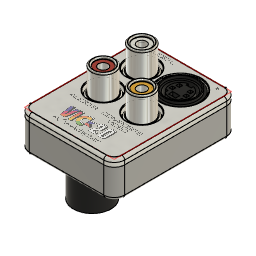
VIC-20_AV_Adapter_case v2 v2 (Autodesk Fusion 360 design; units mm, degrees)
Autodesk Fusion 360 part; units mm, degrees
(part 1 of 2)
sketch "top place" plane through (0, 0, 0) normal (0, 0, 1) x (1, 0, 0) in component "PCB"
  line L0 (0, 1) -> (0, 37)
  circle A0 centre (7, 32) radius 1.7
  arc A1 (23.4749, 22.3133) -> (18.5251, 22.3133) centre (21, 18) ccw
  arc A2 (3.4645, 34.2627) -> (3.4645, 29.7373) centre (7, 32) ccw
  circle A3 centre (21, 18) radius 3.1
  arc A4 (11.3133, 29.5251) -> (11.3133, 34.4749) centre (7, 32) ccw
  arc A5 (16.6867, 20.4749) -> (16.6867, 15.5251) centre (21, 18) ccw
  arc A6 (24.5355, 15.7373) -> (24.5355, 20.2627) centre (21, 18) ccw
  arc A7 (4.5251, 27.6867) -> (9.4749, 27.6867) centre (7, 32) ccw
  arc A8 (11.3133, 15.5251) -> (11.3133, 20.4749) centre (7, 18) ccw
  arc A9 (4.5251, 13.6867) -> (9.4749, 13.6867) centre (7, 18) ccw
  arc A10 (2.6867, 34.4749) -> (2.6867, 29.5251) centre (7, 32) ccw
  arc A11 (10.5355, 29.7373) -> (10.5355, 34.2627) centre (7, 32) ccw
  arc A12 (17.4645, 20.2627) -> (17.4645, 15.7373) centre (21, 18) ccw
  circle A13 centre (7, 18) radius 1.7
  arc A14 (9.2627, 21.5355) -> (4.7373, 21.5355) centre (7, 18) ccw
  arc A15 (4.7373, 21.5355) -> (3.4645, 20.2627) centre (7, 18) ccw
  arc A16 (10.5355, 20.2627) -> (9.2627, 21.5355) centre (7, 18) ccw
  arc A17 (17.4645, 15.7373) -> (18.7373, 14.4645) centre (21, 18) ccw
  arc A18 (2.6867, 29.5251) -> (4.5251, 27.6867) centre (7, 32) ccw
  arc A19 (18.5251, 22.3133) -> (16.6867, 20.4749) centre (21, 18) ccw
  arc A20 (3.4645, 29.7373) -> (4.7373, 28.4645) centre (7, 32) ccw
  arc A21 (18.7373, 21.5355) -> (17.4645, 20.2627) centre (21, 18) ccw
  arc A22 (11.3133, 20.4749) -> (9.4749, 22.3133) centre (7, 18) ccw
  arc A23 (9.2627, 28.4645) -> (10.5355, 29.7373) centre (7, 32) ccw
  arc A24 (9.4749, 13.6867) -> (11.3133, 15.5251) centre (7, 18) ccw
  arc A25 (24.5355, 20.2627) -> (23.2627, 21.5355) centre (21, 18) ccw
  arc A26 (4.5251, 36.3133) -> (2.6867, 34.4749) centre (7, 32) ccw
  arc A27 (3.4645, 15.7373) -> (4.7373, 14.4645) centre (7, 18) ccw
  line L1 (0, 1) -> (0, 38)
  arc A28 (1, 39) -> (0, 38) centre (1, 38) ccw
  arc A29 (29, 38) -> (28, 39) centre (28, 38) ccw
  arc A30 (0, 1) -> (1, 0) centre (1, 1) ccw
  line L2 (28, 0) -> (1, 0)
  line L3 (29, 38) -> (29, 1)
  line L4 (1, 39) -> (28, 39)
  arc A31 (28, 0) -> (29, 1) centre (28, 1) ccw
  circle A32 centre (21, 18) radius 1.7
  arc A33 (9.4749, 36.3133) -> (4.5251, 36.3133) centre (7, 32) ccw
  arc A34 (25.3133, 15.5251) -> (25.3133, 20.4749) centre (21, 18) ccw
  arc A35 (18.5251, 13.6867) -> (23.4749, 13.6867) centre (21, 18) ccw
  arc A36 (18.7373, 14.4645) -> (23.2627, 14.4645) centre (21, 18) ccw
  arc A37 (9.2627, 35.5355) -> (4.7373, 35.5355) centre (7, 32) ccw
  arc A38 (3.4645, 20.2627) -> (3.4645, 15.7373) centre (7, 18) ccw
  line L5 (19.7, 30.5) -> (19.7, 29)
  arc A39 (4.7373, 28.4645) -> (9.2627, 28.4645) centre (7, 32) ccw
  line L6 (21.9, 35) -> (21.9, 35.8)
  circle A40 centre (7, 32) radius 3.1
  line L7 (22.9, 32.2) -> (23.4, 32.2)
  line L8 (20.1, 35) -> (20.1, 35.8)
  arc A41 (9.4749, 22.3133) -> (4.5251, 22.3133) centre (7, 18) ccw
  line L9 (22.3, 29) -> (22.3, 30.5)
  circle A42 centre (7, 18) radius 3.1
  arc A43 (4.7373, 14.4645) -> (9.2627, 14.4645) centre (7, 18) ccw
  arc A44 (10.5355, 15.7373) -> (10.5355, 20.2627) centre (7, 18) ccw
  arc A45 (2.6867, 20.4749) -> (2.6867, 15.5251) centre (7, 18) ccw
  arc A46 (23.2627, 21.5355) -> (18.7373, 21.5355) centre (21, 18) ccw
  line L10 (22.3, 30.5) -> (19.7, 30.5)
  line L11 (19.6, 33) -> (19.6, 34.2)
  line L12 (22.4, 33) -> (22.8, 33)
  line L13 (19.6, 34.2) -> (19.2, 34.2)
  line L14 (19.6, 33) -> (19.2, 33)
  arc A47 (16.2, 31) -> (25.8, 31) centre (21, 32.05) ccw
  arc A48 (25.8, 33) -> (16.2, 33) centre (21, 32) ccw
  line L15 (1.1113, 7.3025) -> (1.4287, 7.62)
  line L16 (3.6513, 8.5725) -> (3.3338, 8.255)
  line L17 (19.1, 32.2) -> (19.1, 31)
  line L18 (20.1, 35) -> (21.9, 35)
  line L19 (3.6513, 7.3025) -> (3.6513, 5.3975)
  line L20 (22.4, 34.2) -> (22.4, 33)
  line L21 (22.9, 31) -> (23.4, 31)
  line L22 (22.4, 34.2) -> (22.8, 34.2)
  line L23 (19.1, 32.2) -> (18.6, 32.2)
  line L24 (19.7, 29) -> (22.3, 29)
  line L25 (22.9, 31) -> (22.9, 32.2)
  line L26 (19.1, 31) -> (18.6, 31)
  circle A49 centre (21, 32) radius 5.6
  line L27 (3.0163, 5.3975) -> (3.6513, 5.3975)
  line L28 (3.6513, 9.8425) -> (3.6513, 8.5725)
  line L29 (1.1113, 6.0325) -> (1.7463, 5.3975)
  line L30 (1.1113, 8.5725) -> (1.1113, 9.8425)
  line L31 (1.1113, 6.0325) -> (1.1113, 7.3025)
  circle A50 centre (21, 32) radius 6
  line L32 (3.0163, 10.4775) -> (3.6513, 9.8425)
  line L33 (3.3338, 7.62) -> (3.6513, 7.3025)
  line L34 (1.7463, 10.4775) -> (3.0163, 10.4775)
  line L35 (1.4287, 8.255) -> (1.1113, 8.5725)
  circle A51 centre (21, 32) radius 6.9
  line L36 (1.7463, 5.3975) -> (3.0163, 5.3975)
  line L37 (1.1113, 9.8425) -> (1.7463, 10.4775)
  line L38 (23.6, 34.2) -> (23.6, 33)
  line L39 (2.6353, 6.4135) -> (2.6353, 6.9215)
  line L40 (17.9, 32.2) -> (17.9, 31)
  arc A52 (25.3133, 20.4749) -> (23.4749, 22.3133) centre (21, 18) ccw
  arc A53 (9.4749, 27.6867) -> (11.3133, 29.5251) centre (7, 32) ccw
  arc A54 (23.2627, 14.4645) -> (24.5355, 15.7373) centre (21, 18) ccw
  line L41 (24.1, 31) -> (24.1, 32.2)
  arc A55 (23.4749, 13.6867) -> (25.3133, 15.5251) centre (21, 18) ccw
  arc A56 (11.3133, 34.4749) -> (9.4749, 36.3133) centre (7, 32) ccw
  line L42 (18.6, 32.2) -> (17.9, 32.2)
  line L43 (22.8, 34.2) -> (23.6, 34.2)
  line L44 (2.6353, 8.9535) -> (2.6353, 9.4615)
  line L45 (2.6353, 9.4615) -> (2.1273, 9.4615)
  line L46 (23.6, 33) -> (22.8, 33)
  arc A57 (4.7373, 35.5355) -> (3.4645, 34.2627) centre (7, 32) ccw
  arc A58 (16.6867, 15.5251) -> (18.5251, 13.6867) centre (21, 18) ccw
  arc A59 (10.5355, 34.2627) -> (9.2627, 35.5355) centre (7, 32) ccw
  arc A60 (2.6867, 15.5251) -> (4.5251, 13.6867) centre (7, 18) ccw
  arc A61 (16.2, 33) -> (16.2, 31) centre (21, 32) ccw
  line L47 (17.9, 31) -> (18.6, 31)
  arc A62 (4.5251, 22.3133) -> (2.6867, 20.4749) centre (7, 18) ccw
  line L48 (23.4, 31) -> (24.1, 31)
  line L49 (19.2, 34.2) -> (18.4, 34.2)
  line L50 (18.4, 33) -> (19.2, 33)
  line L51 (24.1, 32.2) -> (23.4, 32.2)
  line L52 (18.4, 34.2) -> (18.4, 33)
  arc A63 (9.2627, 14.4645) -> (10.5355, 15.7373) centre (7, 18) ccw
  arc A64 (25.8, 31) -> (25.8, 33) centre (21, 32) ccw
  line L53 (1.7463, 7.9375) -> (1.4287, 8.255)
  line L54 (2.1273, 8.9535) -> (2.6353, 8.9535)
  line L55 (3.0163, 7.9375) -> (3.3338, 7.62)
  line L56 (2.1273, 6.4135) -> (2.6353, 6.4135)
  line L57 (2.1273, 9.4615) -> (2.1273, 8.9535)
  line L58 (2.1273, 6.9215) -> (2.1273, 6.4135)
  line L59 (2.6353, 6.9215) -> (2.1273, 6.9215)
  line L60 (1.7463, 7.9375) -> (3.0163, 7.9375)
  line L61 (1.4287, 7.62) -> (1.7463, 7.9375)
  line L62 (3.3338, 8.255) -> (3.0163, 7.9375)
  circle A65 centre (21, 32) radius 4.9031
  line L63 (17.6459, 30) -> (18.5, 30)
  line L64 (20.0999, 35.8) -> (20.1, 35)
  line L65 (20.1, 35) -> (21.9, 35)
  line L66 (21.9, 35) -> (21.9, 35.8)
  circle A66 centre (21, 32) radius 3.9051
  line L67 (18.5, 30) -> (18.5, 29)
  line L68 (23.5, 30) -> (24.3541, 30)
  line L69 (23.5, 30) -> (23.5, 29)
  constraint concentric A48 A65
  constraint equal A48 A65
  constraint perpendicular L6 L65
  constraint coincident L6.end A66
  constraint coincident L63.start A66
  constraint coincident A66 L67.end
  constraint perpendicular L63 L67
  constraint coincident A66 L68.end
  constraint coincident A66 L69.end
  constraint perpendicular L68 L69
extrude "Extrude1" add sketch "top place" against normal blind 1.6 contours L0 L1 A28 A29 A30 L2 L3 L4 A31 | A0 | A1 A5 A19 A34 A35 A52 A55 A58 | A2 A11 A20 A23 A37 A39 A57 A59 | A3 | A4 A7 A10 A18 A26 A33 A53 A56 | A6 A12 A17 A21 A25 A36 A46 A54 | A8 A9 A22 A24 A41 A45 A60 A62 | A13 | A14 A15 A16 A27 A38 A43 A44 A63 | A32 | L5 L9 L10 L24 | L6 L8 L18 L64 L65 L66 A66 | L6 L8 L18 L63 L64 L65 L66 A66 L67 L68 L69 | A66 L68 L69 | L63 A66 L67 | A40 | L7 L21 L25 L41 L48 L51 | A42 | L11 L13 L14 L49 L50 L52 | L12 L20 L22 L38 L43 L46 | A47 A48 A61 A64 A65 | A47 A65 | L15 L19 L27 L29 L31 L33 L36 L55 L60 L61 | L16 L28 L30 L32 L34 L35 L37 L53 L60 L62 | L17 L23 L26 L40 L42 L47 | A49 | A50 | A51 | L39 L56 L58 L59 | L44 L45 L54 L57 makes body 1 in component "PCB"
extrude "Extrude2" add sketch "top place" along normal blind 16.3 contours A3 | A40 | A42 bodies 1 in component "PCB"
extrude "Extrude3" add sketch "top place" along normal blind 17 contours A2 A11 A20 A23 A37 A39 A57 A59 | A6 A12 A17 A21 A25 A36 A46 A54 | A14 A15 A16 A27 A38 A43 A44 A63 bodies 1 in component "PCB"
extrude "Extrude4" add sketch "top place" along normal blind 8 contours A1 A5 A19 A34 A35 A52 A55 A58 | A4 A7 A10 A18 A26 A33 A53 A56 | A8 A9 A22 A24 A41 A45 A60 A62 bodies 1 in component "PCB"
fillet "Fillet3" radius 0.5 9 edges at (3.6119, 20.478, 17) (4.1098, 19.121, 17) (4.522, 28.6119, 17) (4.1098, 33.121, 17) (17.6119, 20.478, 17) (18.1098, 19.121, 17) (10.8671, 14.8735, 8) (24.1265, 21.8671, 8) (3.8735, 28.1329, 8) on bodies 1 in component "PCB"
ref_plane "WorkPlane1" through (0, 0, -1.6) normal (0, 0, 1) x (1, 0, 0) in component "PCB"
sketch "bottom place" plane through (0, 0, -1.6) normal (0, 0, 1) x (1, 0, 0) in component "PCB"
  line L0 (27, 0) -> (1, 0)
  arc A0 (0, 1) -> (1, 0) centre (1, 1) ccw
  circle A1 centre (13, 8) radius 6.8
  arc A2 (11.9, 14.1) -> (14.1, 14.1) centre (13, 14.2) ccw
  circle A3 centre (13, 8) radius 6.2
  circle A4 centre (16.5, 8) radius 0.8
  circle A5 centre (9.5, 8) radius 0.8
  circle A6 centre (15.47, 5.53) radius 0.8
  circle A7 centre (13, 4.5) radius 0.8
  circle A8 centre (10.53, 5.53) radius 0.8
  line L1 (28, 0) -> (1, 0)
  arc A9 (28, 0) -> (29, 1) centre (28, 1) ccw
  line L2 (29, 38) -> (29, 1)
  arc A10 (29, 38) -> (28, 39) centre (28, 38) ccw
  line L3 (1, 39) -> (28, 39)
  arc A11 (1, 39) -> (0, 38) centre (1, 38) ccw
  line L4 (0, 1) -> (0, 38)
extrude "Extrude5" add sketch "bottom place" against normal blind 14.51 contours A4 | A5 | A6 | A7 | A8 bodies 1 in component "PCB"
chamfer "Chamfer1" distance 0.5 angle 45 5 edges at (15.7541, 8.2893, -16.11) (14.7241, 5.8193, -16.11) (12.2541, 4.7893, -16.11) (9.7841, 5.8193, -16.11) (8.7541, 8.2893, -16.11) on bodies 1 in component "PCB"
extrude "Extrude6" add sketch "bottom place" against normal blind 3 from surface at -3 contours A2 A3 | A2 A3 bodies 1 in component "PCB"
extrude "Extrude7" add sketch "bottom place" against normal blind 10 from surface at -5.5 contours A1 bodies 1 in component "PCB"
sketch "bottom stop mask" plane through (0, 0, -1.6) normal (0, 0, 1) x (1, 0, 0) in component "PCB"
  line L0 (27, 0) -> (1, 0)
  line L1 (0, 1) -> (0, 37)
  arc A0 (0, 1) -> (1, 0) centre (1, 1) ccw
  line L2 (14.5294, 4.5894) -> (16.4106, 2.7082)
  line L3 (9.5, 9.3302) -> (6.8396, 9.3302)
  arc A1 (16.5, 9.3302) -> (16.5, 6.6698) centre (16.5, 8) ccw
  line L4 (14.3302, 1.8396) -> (14.3302, 4.5)
  line L5 (16.5, 6.6698) -> (19.1604, 6.6698)
  line L6 (11.6698, 4.5) -> (11.6698, 1.8396)
  line L7 (9.5894, 6.4706) -> (7.7082, 4.5894)
  circle A2 centre (10.5355, 28.4645) radius 1.3716
  circle A3 centre (10.5355, 21.5355) radius 1.3716
  circle A4 centre (7, 18) radius 1.1938
  arc A5 (7.7082, 4.5894) -> (9.5894, 2.7082) centre (8.6488, 3.6488) ccw
  circle A6 centre (17.4645, 14.4645) radius 1.3716
  line L8 (18.2918, 4.5894) -> (16.4106, 6.4706)
  arc A7 (11.4706, 4.5894) -> (9.5894, 6.4706) centre (10.53, 5.53) ccw
  circle A8 centre (3.4645, 14.4645) radius 1.3716
  circle A9 centre (3.4645, 35.5355) radius 1.3716
  line L9 (0, 1) -> (0, 38)
  arc A10 (29, 38) -> (28, 39) centre (28, 38) ccw
  line L10 (28, 0) -> (1, 0)
  arc A11 (0, 1) -> (1, 0) centre (1, 1) ccw
  line L11 (29, 38) -> (29, 1)
  arc A12 (1, 39) -> (0, 38) centre (1, 38) ccw
  line L12 (1, 39) -> (28, 39)
  arc A13 (28, 0) -> (29, 1) centre (28, 1) ccw
  line L13 (1.4669, 5.7531) -> (3.2957, 5.7531)
  circle A14 centre (7, 32) radius 1.1938
  circle A15 centre (3.4645, 21.5355) radius 1.3716
  circle A16 centre (24.5355, 14.4645) radius 1.3716
  circle A17 centre (17.4645, 21.5355) radius 1.3716
  arc A18 (19.1604, 6.6698) -> (19.1604, 9.3302) centre (19.1604, 8) ccw
  line L14 (19.1604, 9.3302) -> (16.5, 9.3302)
  circle A19 centre (24.5355, 21.5355) radius 1.3716
  circle A20 centre (21, 18) radius 1.1938
  arc A21 (14.3302, 4.5) -> (11.6698, 4.5) centre (13, 4.5) ccw
  circle A22 centre (18.6, 33.6) radius 0.8302
  circle A23 centre (25.6, 32) radius 0.9302
  arc A24 (9.5, 6.6698) -> (9.5, 9.3302) centre (9.5, 8) ccw
  line L15 (3.2957, 5.7531) -> (3.2957, 7.5819)
  circle A25 centre (3.4645, 28.4645) radius 1.3716
  circle A26 centre (10.5355, 14.4645) radius 1.3716
  arc A27 (6.8396, 9.3302) -> (6.8396, 6.6698) centre (6.8396, 8) ccw
  arc A28 (16.4106, 6.4706) -> (14.5294, 4.5894) centre (15.47, 5.53) ccw
  circle A29 centre (10.5355, 35.5355) radius 1.3716
  line L16 (3.2957, 7.5819) -> (1.4669, 7.5819)
  line L17 (9.5894, 2.7082) -> (11.4706, 4.5894)
  arc A30 (11.6698, 1.8396) -> (14.3302, 1.8396) centre (13, 1.8396) ccw
  line L18 (6.8396, 6.6698) -> (9.5, 6.6698)
  arc A31 (16.4106, 2.7082) -> (18.2918, 4.5894) centre (17.3512, 3.6488) ccw
  line L19 (1.4669, 7.5819) -> (1.4669, 5.7531)
  circle A32 centre (2.3813, 9.2075) radius 0.9144
  circle A33 centre (23.9, 31.6) radius 0.8302
  circle A34 centre (18.1, 31.6) radius 0.8302
  circle A35 centre (23.4, 33.6) radius 0.8302
  circle A36 centre (16.4, 32) radius 0.9302
extrude "Extrude8" add sketch "bottom stop mask" against normal blind 1.5 contours A2 | A3 | A4 | A6 | A8 | A9 | L13 L15 L16 L19 | A14 | A15 | A16 | A17 | A19 | A20 | A22 | A23 A33 | A23 A33 | A25 | A26 | A29 | A32 | A34 A36 | A34 A36 | A35 picked at (25.9085, 32.0541) picked at (23.634, 31.5105) picked at (18.3763, 31.5534) picked at (16.1011, 32.0945) bodies 1 in component "PCB"
chamfer "Chamfer3" distance 0.5 angle 45 20 edges at (1.4669, 6.6675, -3.1) (2.3813, 7.5819, -3.1) (3.2957, 6.6675, -3.1) (2.3813, 5.7531, -3.1) (1.5288, 9.5382, -3.1) (2.1857, 14.9605, -3.1) (5.887, 18.4317, -3.1) (2.1857, 22.0315, -3.1) (9.2567, 14.9605, -3.1) (9.2567, 22.0315, -3.1) (2.1857, 28.9605, -3.1) (2.1857, 36.0315, -3.1) (5.887, 32.4317, -3.1) (9.2567, 28.9605, -3.1) (9.2567, 36.0315, -3.1) (23.2567, 22.0315, -3.1) (16.1857, 22.0315, -3.1) (19.887, 18.4317, -3.1) (23.2567, 14.9605, -3.1) (16.1857, 14.9605, -3.1) on bodies 1 in component "PCB"
extrude "Extrude10" add sketch "top place" along normal blind 1 from surface at 7.5 separate body contours A51 makes body 2 in component "PCB"
extrude "Extrude11" add sketch "top place" along normal blind 9.5 contours A50 bodies 2 1 in component "PCB"
extrude "Extrude12" add sketch "top place" along normal blind 8.5 separate body contours L6 L8 L18 L63 L64 L65 L66 A66 L67 L68 L69 makes body 3 in component "PCB"
extrude "Extrude13" add sketch "top place" along normal blind 8.5 separate body contours A49 makes body 4 in component "PCB"
combine "Combine1" operation add target body 2 tool bodies 3 4 in component "PCB"
ref_plane "WorkPlane1" through (14.5, 19.5, -1.7) normal (0, 0, -1) x (-1, 0, 0) in component "bottom shell"
sketch "bottom shell base" plane through (14, 19, -1.7) normal (0, 0, -1) x (1, 0, 0) in component "bottom shell"
  circle A0 centre (-1, 11) radius 6.8 construction
  line L0 (-14.3, 18) -> (-14.3, -19)
  arc A1 (-14.3, -19) -> (-13, -20.3) centre (-13, -19) ccw
  line L1 (-13, -20.3) -> (14, -20.3)
  arc A2 (14, -20.3) -> (15.3, -19) centre (14, -19) ccw
  line L2 (15.3, -19) -> (15.3, 18)
  arc A3 (15.3, 18) -> (14, 19.3) centre (14, 18) ccw
  line L3 (14, 19.3) -> (-13, 19.3)
  arc A4 (-13, 19.3) -> (-14.3, 18) centre (-13, 18) ccw
  circle A5 centre (-1, 11) radius 7.1
  line L4 (-13, -22.8) -> (14, -22.8)
  arc A6 (14, -22.8) -> (17.8, -19) centre (14, -19) ccw
  line L5 (17.8, -19) -> (17.8, 18)
  arc A7 (17.8, 18) -> (14, 21.8) centre (14, 18) ccw
  line L6 (14, 21.8) -> (-13, 21.8)
  arc A8 (-13, 21.8) -> (-16.8, 18) centre (-13, 18) ccw
  line L7 (-16.8, 18) -> (-16.8, -19)
  arc A9 (-16.8, -18.996) -> (-13, -22.8) centre (-13, -19) ccw
  line L8 (-13, -21.8) -> (14, -21.8)
  line L9 (16.8, -19) -> (16.8, 18)
  arc A10 (16.8, 18) -> (14, 20.8) centre (14, 18) ccw
  line L10 (14, 20.8) -> (-13, 20.8)
  arc A11 (-13, 20.8) -> (-15.8, 18) centre (-13, 18) ccw
  line L11 (-15.8, 18) -> (-15.8, -19)
  arc A12 (-15.8, -19) -> (-13, -21.8) centre (-13, -19) ccw
  line L12 (-14, 18) -> (-14, -19) construction
  arc A13 (-13, 19) -> (-14, 18) centre (-13, 18) ccw construction
  line L13 (14, 19) -> (-13, 19) construction
  arc A14 (15, 18) -> (14, 19) centre (14, 18) ccw construction
  line L14 (15, -19) -> (15, 18) construction
  arc A15 (14, -20) -> (15, -19) centre (14, -19) ccw construction
  line L15 (-13, -20) -> (14, -20) construction
  arc A16 (-14, -19) -> (-13, -20) centre (-13, -19) ccw construction
  line L16 (-14, -19) -> (-16.8, -19) construction
  line L17 (-13, -20) -> (-13, -22.8) construction
  line L18 (14, -20) -> (14, -22.8) construction
  line L19 (15, -19) -> (17.8, -19) construction
  arc A17 (14, -21.8) -> (16.8, -19) centre (14, -19) ccw
  line L20 (14, 19) -> (14, 22.99) construction
  line L21 (15, 18) -> (19.6847, 18) construction
  line L22 (-13, 19) -> (-13, 21.8) construction
  line L23 (-14, 18) -> (-16.8, 18) construction
  dimension "d28" = 0.3
  dimension "d177" = 0.3
  dimension "d178" = 0.3
  dimension "d179" = 0.3
  dimension "d180" = 0.3
  dimension "d182" = 2.8
  dimension "d183" = 2.8
  dimension "d189" = 1.8
  dimension "d190" = 1.8
  dimension "d191" = 1.8
  dimension "d192" = 1.8
  dimension "d193" = 1.8
  dimension "d194" = 1.8
  dimension "d195" = 1.8
  dimension "d198" = 2.8
  dimension "d199" = 2.8
  constraint tangent A1 L1
  constraint tangent A2 L2
  constraint tangent L1 A2
  constraint tangent L2 A3
  constraint tangent A3 L3
  constraint concentric A1 A16
  constraint concentric A2 A15
  constraint concentric A3 A14
  constraint parallel L9 L14
  constraint parallel L10 L13
  constraint parallel L8 L15
  constraint concentric A4 A13
  constraint concentric A11 A13
  constraint concentric A1 A12
  constraint concentric A10 A14
  constraint concentric A9 A16
  constraint coincident L12.end A16.start
  constraint perpendicular L7 L16
  constraint coincident L15.start A16.end
  constraint perpendicular L4 L17
  constraint coincident A15.start L15.end
  constraint perpendicular L4 L18
  constraint coincident L14.start A15.end
  constraint perpendicular L5 L19
  constraint coincident L7 L16.end
  constraint concentric A2 A17
  constraint tangent L8 A17
  constraint tangent L4 A6
  constraint tangent A7 L6
  constraint coincident L13.start A14.end
  constraint perpendicular L6 L20
  constraint coincident A14.start L14.end
  constraint perpendicular L2 L21
  constraint coincident A7.end L20
  constraint coincident L5.end L21
  constraint coincident A13.start L13.end
  constraint perpendicular L10 L22
  constraint coincident L12.start A13.end
  constraint perpendicular L0 L23
  constraint tangent A8 L7
  measures "d177" distance of L0 L12
  measures "d178" distance of L3 L13
  measures "d179" distance of L1 L15
  measures "d180" distance of L2 L14
  measures "d182" distance of L7 L12
  measures "d183" distance of L6 L13
  measures "d189" distance of L11 L12
  measures "d190" distance of L10 L13
  measures "d191" distance of L9 L14
  measures "d192" distance of L8 L15
  measures "d193" distance of A12 A16
  measures "d194" distance of A11 A13
  measures "d195" distance of A10 A14
  measures "d198" distance of L4 L15
  measures "d199" distance of L5 L14
extrude "Extrude1'" add sketch "bottom shell base" along normal blind 2.5 separate body contours L0 A1 L1 A2 L2 A3 L3 A4 | L4 A6 L5 A7 L6 A8 L7 A9 | L8 L9 A10 L10 A11 L11 A12 A17 makes body 5 in component "bottom shell"
sketch "solder pads v1" plane through (0, 0, -1.7) normal (0, 0, 1) x (-1, 0, 0) in component "bottom shell"
  circle A0 centre (-13, -8) radius 7.1
  line L0 (-1, 2.8) -> (-28, 2.8)
  arc A1 (-28, 2.8) -> (-31.8, -1) centre (-28, -1) ccw
  line L1 (-31.8, -1) -> (-31.8, -38)
  arc A2 (-31.8, -38) -> (-28, -41.8) centre (-28, -38) ccw
  line L2 (-28, -41.8) -> (-1, -41.8)
  circle A3 centre (-23.4, -33.6) radius 0.8302 construction
  circle A4 centre (-23.9, -31.6) radius 0.8302 construction
  circle A5 centre (-25.6, -32) radius 0.9302 construction
  circle A6 centre (-18.1, -31.6) radius 0.8302 construction
  circle A7 centre (-16.4, -32) radius 0.9302 construction
  circle A8 centre (-18.6, -33.6) radius 0.8302 construction
  line L3 (-15.6019, -33.1868) -> (-17.8577, -34.7038)
  line L4 (-19.3905, -31.2774) -> (-19.8905, -33.2774)
  line L5 (-16.1527, -30.5913) -> (-17.87, -30.2898)
  arc A9 (-15.6019, -33.1868) -> (-16.1527, -30.5913) centre (-16.4, -32) ccw
  arc A10 (-17.87, -30.2898) -> (-19.3905, -31.2774) centre (-18.1, -31.6) ccw
  arc A11 (-19.8905, -33.2774) -> (-17.8577, -34.7038) centre (-18.6, -33.6) ccw
  line L6 (-22.1095, -33.2774) -> (-22.6095, -31.2774)
  line L7 (-24.13, -30.2898) -> (-25.8473, -30.5913)
  line L8 (-24.1423, -34.7038) -> (-26.3981, -33.1868)
  arc A12 (-24.1423, -34.7038) -> (-22.1095, -33.2774) centre (-23.4, -33.6) ccw
  arc A13 (-23.9862, -32.406) -> (-24.0175, -32.4218) centre (-23.4, -33.6) ccw
  arc A14 (-22.6095, -31.2774) -> (-24.13, -30.2898) centre (-23.9, -31.6) ccw
  arc A15 (-25.8473, -30.5913) -> (-26.3981, -33.1868) centre (-25.6, -32) ccw
  arc A16 (-23.9912, -32.4252) -> (-23.9862, -32.406) centre (-25.6, -32) ccw
  dimension "d215" = 0.5
  dimension "d216" = 0.5
  dimension "d217" = 0.5
  dimension "d218" = 0.5
  dimension "d219" = 0.5
  dimension "d220" = 0.5
  constraint concentric A7 A9
  constraint concentric A6 A10
  constraint concentric A8 A11
  constraint concentric A3 A12
  constraint concentric A5 A15
  constraint tangent L5 A9
  constraint tangent L5 A10
  constraint tangent L3 A11
  constraint tangent L3 A9
  constraint tangent L4 A10
  constraint tangent L4 A11
  constraint tangent L6 A12
  constraint tangent L7 A15
  constraint tangent L8 A15
  constraint tangent L8 A12
  constraint coincident A13.start A12
  constraint coincident A4 A13.end
  constraint concentric A12 A13
  constraint coincident A4 A16.start
  constraint concentric A15 A16
  constraint tangent L6 A14
  constraint tangent L7 A14
  measures "d215" distance of A7 A9
  measures "d216" distance of A6 A10
  measures "d217" distance of A8 A11
  measures "d218" distance of A4 A14
  measures "d219" distance of A3 A12
  measures "d220" distance of A5 A15
sketch "Sketch9" plane through (0, 0, -1.7) normal (0, 0, 1) x (-1, 0, 0) in component "bottom shell"
  circle A0 centre (-13, -8) radius 7.1
  arc A1 (-1, -41.8) -> (2.8, -37.996) centre (-1, -38) ccw
  line L0 (2.8, -37.996) -> (2.8, -1)
  arc A2 (2.8, -1) -> (-1, 2.8) centre (-1, -1) ccw
  line L1 (-1, 2.8) -> (-28, 2.8)
  arc A3 (-28, 2.8) -> (-31.8, -1) centre (-28, -1) ccw
  line L2 (-31.8, -1) -> (-31.8, -38)
  arc A4 (-31.8, -38) -> (-28, -41.8) centre (-28, -38) ccw
  line L3 (-28, -41.8) -> (-1, -41.8)
  line L4 (-0.9929, -38.9571) -> (-27.9929, -38.9571)
  arc A5 (-28.9929, -37.9571) -> (-27.9929, -38.9571) centre (-27.9929, -37.9571) ccw
  line L5 (-28.9929, -37.9571) -> (-28.9929, -0.9571)
  line L6 (-27.9929, 0.0429) -> (-0.9929, 0.0429)
  arc A6 (-27.9929, 0.0429) -> (-28.9929, -0.9571) centre (-27.9929, -0.9571) ccw
  line L7 (0.0071, -0.9571) -> (0.0071, -37.9571)
  arc A7 (-0.9929, -38.9571) -> (0.0071, -37.9571) centre (-0.9929, -37.9571) ccw
  arc A8 (0.0071, -0.9571) -> (-0.9929, 0.0429) centre (-0.9929, -0.9571) ccw
  circle A9 centre (-3.3513, -14.3155) radius 1.3716 construction
  circle A10 centre (-5.8615, -19.0885) radius 1.3516 construction
  circle A11 centre (-25.5929, -31.9571) radius 0.9302
  circle A12 centre (-16.3929, -31.9571) radius 0.9302
  circle A13 centre (-10.6345, -21.5987) radius 1.3716 construction
  circle A14 centre (-23.3929, -33.5571) radius 0.8302
  circle A15 centre (-18.0929, -31.5571) radius 0.8302
  circle A16 centre (-5.8615, -33.0885) radius 1.3516 construction
  circle A17 centre (-24.6345, -14.3155) radius 1.3716 construction
  line L8 (-18.2847, -4.5465) -> (-16.4035, -6.4277)
  line L9 (-19.1533, -9.2873) -> (-16.4929, -9.2873)
  arc A18 (-16.4035, -6.4277) -> (-14.5224, -4.5465) centre (-15.4629, -5.4871) ccw
  arc A19 (-11.4635, -4.5465) -> (-9.5824, -6.4277) centre (-10.5229, -5.4871) ccw
  arc A20 (-7.7012, -4.5465) -> (-9.5824, -2.6653) centre (-8.6418, -3.6059) ccw
  arc A21 (-14.3231, -4.4571) -> (-11.6627, -4.4571) centre (-12.9929, -4.4571) ccw
  line L10 (-14.3231, -1.7967) -> (-14.3231, -4.4571)
  line L11 (-9.5824, -6.4277) -> (-7.7012, -4.5465)
  arc A22 (-16.4929, -9.2873) -> (-16.4929, -6.6269) centre (-16.4929, -7.9571) ccw
  line L12 (-16.4929, -6.6269) -> (-19.1533, -6.6269)
  arc A23 (-9.4929, -6.6269) -> (-9.4929, -9.2873) centre (-9.4929, -7.9571) ccw
  arc A24 (-16.4035, -2.6653) -> (-18.2847, -4.5465) centre (-17.3441, -3.6059) ccw
  line L13 (-6.8325, -6.6269) -> (-9.4929, -6.6269)
  arc A25 (-11.6627, -1.7967) -> (-14.3231, -1.7967) centre (-12.9929, -1.7967) ccw
  line L14 (-11.6627, -4.4571) -> (-11.6627, -1.7967)
  circle A26 centre (-10.6345, -35.5987) radius 1.3716 construction
  line L15 (-9.5824, -2.6653) -> (-11.4635, -4.5465)
  arc A27 (-6.8325, -9.2873) -> (-6.8325, -6.6269) centre (-6.8325, -7.9571) ccw
  line L16 (-14.5224, -4.5465) -> (-16.4035, -2.6653)
  circle A28 centre (-22.1243, -19.0885) radius 1.3516 construction
  line L17 (-9.4929, -9.2873) -> (-6.8325, -9.2873)
  circle A29 centre (-17.3513, -21.5987) radius 1.3716 construction
  circle A30 centre (-3.3513, -28.3155) radius 1.3716 construction
  arc A31 (-19.1533, -6.6269) -> (-19.1533, -9.2873) centre (-19.1533, -7.9571) ccw
  circle A32 centre (-18.5929, -33.5571) radius 0.8302
  circle A33 centre (-23.8929, -31.5571) radius 0.8302
  circle A34 centre (-24.6345, -14.3155) radius 1.6716
  circle A35 centre (-22.1243, -19.0885) radius 1.6516
  circle A36 centre (-17.3513, -21.5987) radius 1.6716
  circle A37 centre (-10.6345, -21.5987) radius 1.6716
  circle A38 centre (-5.8615, -19.0885) radius 1.6516
  circle A39 centre (-3.3513, -14.3155) radius 1.6716
  circle A40 centre (-3.3513, -28.3155) radius 1.6716
  circle A41 centre (-5.8615, -33.0885) radius 1.6516
  circle A42 centre (-10.6345, -35.5987) radius 1.6716
  dimension "d237" = 0.3
  dimension "d238" = 0.3
  dimension "d239" = 0.3
  dimension "d240" = 0.3
  dimension "d241" = 0.3
  dimension "d242" = 0.3
  dimension "d243" = 0.3
  dimension "d244" = 0.3
  dimension "d245" = 0.3
extrude "Extrude2'" cut sketch "solder pads v1" sketch "Sketch9" against normal blind 1.5 contours L3 L4 L5 A9 A10 A11 | L6 L7 L8 A12 A14 A15 of sketch 2 contours A34 | A35 | A36 | A37 | A38 | A39 | A40 | A41 | A42 bodies 5 in component "bottom shell"
extrude "Extrude3'" add sketch "bottom shell base" against normal blind 6.5 contours L8 L9 A10 L10 A11 L11 A12 A17 bodies 5 in component "bottom shell"
extrude "Extrude4'" add sketch "bottom shell base" against normal blind 8 contours L4 A6 L5 A7 L6 A8 L7 A9 bodies 5 in component "bottom shell"
fillet "Fillet1" radius 1 8 edges at (14.5, 41.8, -4.2) (30.687, 40.687, -4.2) (31.8, 19.5, -4.2) (30.687, -1.687, -4.2) (14.5, -2.8, -4.2) (-1.687, -1.687, -4.2) (-2.8, 19.498, -4.2) (-1.6884, 40.6856, -4.2) on bodies 5 in component "bottom shell"
ref_plane "WorkPlane1" through (30.8, -2.8, 6.3) normal (0, 0, 1) x (1, 0, 0) in component "top shell"
sketch "top shell" plane through (29.5, -2.3, 6.3) normal (0, 0, 1) x (1, 0, 0) in component "top shell"
  arc A0 (-32.3, 3.3) -> (-28.5, -0.5) centre (-28.5, 3.3) ccw
  line L0 (-32.3, 40.296) -> (-32.3, 3.3)
  arc A1 (-28.5, 44.1) -> (-32.3, 40.296) centre (-28.5, 40.3) ccw
  line L1 (-1.5, 44.1) -> (-28.5, 44.1)
  arc A2 (2.3, 40.3) -> (-1.5, 44.1) centre (-1.5, 40.3) ccw
  line L2 (2.3, 3.3) -> (2.3, 40.3)
  arc A3 (-1.5, -0.5) -> (2.3, 3.3) centre (-1.5, 3.3) ccw
  line L3 (-28.5, -0.5) -> (-1.5, -0.5)
  line L4 (-29.8, 3.3) -> (-29.8, 40.3)
  arc A4 (-29.8, 3.3) -> (-28.5, 2) centre (-28.5, 3.3) ccw
  line L5 (-1.5, 2) -> (-28.5, 2)
  arc A5 (-28.5, 41.6) -> (-29.8, 40.3) centre (-28.5, 40.3) ccw
  line L6 (-28.5, 41.6) -> (-1.5, 41.6)
  arc A6 (-0.2, 40.3) -> (-1.5, 41.6) centre (-1.5, 40.3) ccw
  line L7 (-0.2, 40.3) -> (-0.2, 3.3)
  arc A7 (-1.5, 2) -> (-0.2, 3.3) centre (-1.5, 3.3) ccw
  arc A8 (-26.8133, 31.8251) -> (-24.9749, 29.9867) centre (-22.5, 34.3) ccw construction
  arc A9 (-18.1867, 31.8251) -> (-18.1867, 36.7749) centre (-22.5, 34.3) ccw construction
  arc A10 (-24.9749, 38.6133) -> (-26.8133, 36.7749) centre (-22.5, 34.3) ccw construction
  arc A11 (-28.5, 42.6) -> (-30.8, 40.3) centre (-28.5, 40.3) ccw
  line L8 (-30.8, 3.3) -> (-30.8, 40.3)
  arc A12 (-30.8, 3.3) -> (-28.5, 1) centre (-28.5, 3.3) ccw
  line L9 (-1.5, 1) -> (-28.5, 1)
  arc A13 (-1.5, 1) -> (0.8, 3.3) centre (-1.5, 3.3) ccw
  line L10 (0.8, 40.3) -> (0.8, 3.3)
  arc A14 (0.8, 40.3) -> (-1.5, 42.6) centre (-1.5, 40.3) ccw
  line L11 (-28.5, 42.6) -> (-1.5, 42.6)
  circle A15 centre (-16.5, 10.3) radius 6.8 construction
  circle A16 centre (-16.5, 10.3) radius 2
  line L12 (-29.8, 6) -> (-27.3, 6)
  line L13 (-27.3, 6) -> (-27.3, 14)
  line L14 (-27.3, 14) -> (-29.8, 14)
  line L15 (-29.8, 14) -> (-29.8, 6)
  line L16 (-8.7, 2) -> (-16.7, 2)
  line L17 (-16.7, 2) -> (-16.7, 4.5)
  line L18 (-16.7, 4.5) -> (-8.7, 4.5)
  line L19 (-8.7, 4.5) -> (-8.7, 2)
  line L20 (-19.5, 41.6) -> (-14.7, 41.6)
  line L21 (-14.7, 41.6) -> (-14.7, 39.1)
  line L22 (-14.7, 39.1) -> (-19.5, 39.1)
  line L23 (-19.5, 39.1) -> (-19.5, 41.6)
  line L24 (-0.2, 14) -> (-2.7, 14)
  line L25 (-2.7, 14) -> (-2.7, 6)
  line L26 (-2.7, 6) -> (-0.2, 6)
  line L27 (-0.2, 6) -> (-0.2, 14)
  circle A17 centre (-22.5, 34.3) radius 4.9729 construction
  circle A18 centre (-8.5, 34.3) radius 6.9 construction
  arc A19 (-24.9749, 24.6133) -> (-26.8133, 22.7749) centre (-22.5, 20.3) ccw construction
  arc A20 (-10.9749, 24.6133) -> (-12.8133, 22.7749) centre (-8.5, 20.3) ccw construction
  arc A21 (-12.8133, 17.8251) -> (-10.9749, 15.9867) centre (-8.5, 20.3) ccw construction
  arc A22 (-18.1867, 17.8251) -> (-18.1867, 22.7749) centre (-22.5, 20.3) ccw construction
  arc A23 (-26.8133, 17.8251) -> (-24.9749, 15.9867) centre (-22.5, 20.3) ccw construction
  arc A24 (-4.1867, 17.8251) -> (-4.1867, 22.7749) centre (-8.5, 20.3) ccw construction
  circle A25 centre (-22.5, 20.3) radius 4.9729 construction
  circle A26 centre (-8.5, 20.3) radius 4.9729 construction
  circle A27 centre (-22.5, 34.3) radius 5.4729
  circle A28 centre (-22.5, 20.3) radius 5.4729
  circle A29 centre (-8.5, 20.3) radius 5.4729
  circle A30 centre (-8.5, 34.3) radius 7.3
  dimension "d64" = 1
  dimension "d65" = 4
  dimension "d69" = 2.5
  dimension "d70" = 8
  dimension "d71" = 4
  dimension "d72" = 8
  dimension "d73" = 2.5
  dimension "d74" = 8.5
  dimension "d75" = 4.8
  dimension "d76" = 2.5
  dimension "d78" = 2.5
  dimension "d79" = 8
  dimension "d222" = 0.5
  dimension "d223" = 0.5
  dimension "d224" = 0.5
  dimension "d226" = 3
  constraint concentric A15 A16
  constraint horizontal L12
  constraint vertical L13
  constraint horizontal L14
  constraint vertical L15
  constraint coincident L4 L12.start
  constraint horizontal L16
  constraint vertical L17
  constraint horizontal L18
  constraint vertical L19
  constraint coincident L5 L16.start
  constraint horizontal L20
  constraint vertical L21
  constraint horizontal L22
  constraint vertical L23
  constraint coincident L6 L20.start
  constraint horizontal L24
  constraint vertical L25
  constraint horizontal L26
  constraint vertical L27
  constraint coincident L7 L24.start
  constraint collinear L14 L24
  constraint coincident A10.end A17
  constraint coincident A9.end A17
  constraint coincident A8.end A17
  constraint coincident A19.start A25
  constraint coincident A23.end A25
  constraint coincident A22.end A25
  constraint coincident A20.end A26
  constraint coincident A21.end A26
  constraint coincident A24.end A26
  constraint concentric A17 A27
  constraint concentric A25 A28
  constraint concentric A24 A29
  constraint concentric A18 A30
  constraint tangent L6 A30
  measures "d65" diameter of A16
  measures "d69" distance of L12.start L12.end
  measures "d70" distance of L12.start L14.end
  measures "d71" distance of L5 L12
  measures "d72" distance of L16.start L16.end
  measures "d73" distance of L16.start L18.end
  measures "d74" distance of L7 L19
  measures "d75" distance of L20.start L20.end
  measures "d76" distance of L20.start L22.end
  measures "d78" distance of L24.start L24.end
  measures "d79" distance of L24.start L26.end
  measures "d222" distance of A17 A27
  measures "d223" distance of A25 A28
  measures "d224" distance of A26 A29
  measures "d226" distance of A8.centre L23
extrude "Extrude1''" add sketch "top shell" along normal blind 2.5 separate body contours A0 L0 A1 L1 A2 L2 A3 L3 | L4 A4 L5 A5 L6 A6 L7 A7 L12 L13 L14 L17 L18 L19 L21 L22 L23 L24 L25 L26 | L4 L12 L13 L14 L15 | L5 L16 L17 L18 L19 | L6 L20 L21 L22 L23 | L7 L24 L25 L26 L27 | A11 L8 A12 L9 A13 L10 A14 L11 | A16 makes body 6 in component "top shell"
extrude "Extrude2''" add sketch "top shell" against normal blind 1.5 contours A11 L8 A12 L9 A13 L10 A14 L11 bodies 6 in component "top shell"
extrude "Extrude3''" add sketch "top shell" against normal blind 6 draft -7 contours A16 bodies 6 in component "top shell"
extrude "Extrude4''" add sketch "top shell" against normal blind 6 contours L4 L12 L13 L14 L15 | L5 L16 L17 L18 L19 | L6 L20 L21 L22 L23 | L7 L24 L25 L26 L27 bodies 6 in component "top shell"
sketch "bot_hook" plane through (12.8, 0, 0) normal (-1, 0, 0) x (0, -1, 0) in component "top shell"
  line L0 (0.3, 6.3) -> (-2.2, 6.3)
  line L1 (-2.2, 6.3) -> (-2.2, 0.3)
  line L2 (-2.2, 0.3) -> (0.3, 0.3)
  line L3 (0.3, 0.3) -> (0.3, 4.8)
  line L4 (0.3, 4.8) -> (0.3, 6.3)
  line L5 (0.3, 0.3) -> (-2.2, 0.3) construction
  line L6 (0.3, 4.8) -> (0.3, 0.3) construction
  line L7 (0.3, 0.3) -> (1.1, 2.7374)
  line L8 (1.1, 2.7374) -> (0.3, 3)
  line L9 (0.3, 0.3) -> (0.3, 3)
  dimension "d95" = 0.8
  dimension "d96" = 2.7
  constraint coincident L2.end L3.start
  constraint coincident L3 L8.end
  constraint perpendicular L7 L8
  measures "d95" horizontal distance of L2.end L7.end
  measures "d96" distance of L2.end L8.end
sketch "left_hook" plane through (0, 3.7, 0) normal (0, -1, 0) x (1, 0, 0) in component "top shell"
  line L0 (29.3, 6.3) -> (26.8, 6.3)
  line L1 (26.8, 6.3) -> (26.8, 0.3)
  line L2 (26.8, 0.3) -> (29.3, 0.3)
  line L3 (29.3, 0.3) -> (29.3, 4.8)
  line L4 (29.3, 4.8) -> (29.3, 6.3)
  line L5 (29.3, 0.3) -> (26.8, 0.3) construction
  line L6 (29.3, 4.8) -> (29.3, 0.3) construction
  line L7 (29.3, 0.3) -> (30.1, 2.7374)
  line L8 (30.1, 2.7374) -> (29.3, 3)
  line L9 (29.3, 3) -> (29.3, 0.3)
  dimension "d97" = 0.8
  dimension "d98" = 2.7
  constraint coincident L2.end L3.start
  constraint coincident L3 L8.end
  constraint perpendicular L7 L8
  measures "d97" distance of L3 L7.end
  measures "d98" distance of L8.end L2.end
sketch "right_hook" plane through (0, 11.7, 0) normal (0, 1, 0) x (-1, 0, 0) in component "top shell"
  line L0 (0.3, 6.3) -> (-2.2, 6.3)
  line L1 (-2.2, 6.3) -> (-2.2, 0.3)
  line L2 (-2.2, 0.3) -> (0.3, 0.3)
  line L3 (0.3, 0.3) -> (0.3, 4.8)
  line L4 (0.3, 4.8) -> (0.3, 6.3)
  line L5 (0.3, 0.3) -> (-2.2, 0.3) construction
  line L6 (0.3, 4.8) -> (0.3, 0.3) construction
  line L7 (0.3, 0.3) -> (1.1, 2.7374)
  line L8 (1.1, 2.7374) -> (0.3, 3)
  line L9 (0.3, 3) -> (0.3, 0.3)
  dimension "d99" = 2.7
  dimension "d100" = 0.8
  constraint coincident L2.end L3.start
  constraint coincident L6 L8.end
  constraint perpendicular L7 L8
  measures "d99" distance of L2.end L8.end
  measures "d100" distance of L7.end L9
sketch "top_hook" plane through (10, 0, 0) normal (-1, 0, 0) x (0, -1, 0) in component "top shell"
  line L0 (-36.8, 6.3) -> (-39.3, 6.3)
  line L1 (-39.3, 6.3) -> (-39.3, 4.8)
  line L2 (-39.3, 4.8) -> (-39.3, 0.3)
  line L3 (-39.3, 0.3) -> (-36.8, 0.3)
  line L4 (-36.8, 0.3) -> (-36.8, 6.3)
  line L5 (-36.8, 0.3) -> (-39.3, 0.3) construction
  line L6 (-39.3, 4.8) -> (-39.3, 0.3) construction
  line L7 (-39.3, 0.3) -> (-40.1, 2.7374)
  line L8 (-40.1, 2.7374) -> (-39.3, 3)
  line L9 (-39.3, 3) -> (-39.3, 0.3)
  dimension "d101" = 2.7
  dimension "d102" = 0.8
  constraint coincident L2.end L3.start
  constraint coincident L6 L8.end
  constraint perpendicular L7 L8
  measures "d101" distance of L8.end L2.end
  measures "d102" distance of L7.end L9
extrude "Extrude5'" add sketch "top_hook" against normal blind 4.8 contours L2 L7 L8 L9 bodies 6 in component "top shell"
extrude "Extrude6'" add sketch "left_hook" against normal blind 8 contours L3 L7 L8 L9 bodies 6 in component "top shell"
extrude "Extrude7'" add sketch "bot_hook" against normal blind 8 contours L3 L7 L8 L9 bodies 6 in component "top shell"
extrude "Extrude8'" add sketch "right_hook" against normal blind 8 contours L3 L7 L8 L9 bodies 6 in component "top shell"
sketch "left" plane through (-0.3, 0, 0) normal (1, 0, 0) x (0, 1, 0) in component "bottom shell"
  line L0 (1, -1.7) -> (38, -1.7)
  line L1 (38, -1.7) -> (38, 4.8)
  line L2 (38, 4.8) -> (1, 4.8)
  line L3 (1, 4.8) -> (1, -1.7)
  line L4 (3.7, 0.3) -> (11.7, 0.3) construction
  line L5 (3.7, 6.3) -> (3.7, 0.3) construction
  line L6 (11.7, 6.3) -> (11.7, 0.3) construction
  line L7 (11.7, 0.3) -> (11.7, 2.7374) construction
  line L8 (11.7, 2.7374) -> (11.7, 3) construction
  line L9 (11.7, 3) -> (11.7, 4.8) construction
  line L10 (11.7, 4.8) -> (11.7, 6.3) construction
  line L11 (11.7, 3) -> (3.7, 3) construction
  line L12 (3.4, 6.3) -> (12, 6.3)
  line L13 (12, 6.3) -> (12, 0)
  line L14 (12, 0) -> (3.4, 0)
  line L15 (3.4, 0) -> (3.4, 6.3)
  line L16 (3.4, 3.3) -> (12, 3.3)
  line L17 (1, -1.7) -> (38, -1.7)
  line L18 (38, -1.7) -> (38, 4.8)
  line L19 (38, 4.8) -> (1, 4.8)
  line L20 (1, 4.8) -> (1, -1.7)
  dimension "d113" = 0.3
  dimension "d114" = 0.3
  dimension "d115" = 0.3
  dimension "d116" = 0.3
  constraint horizontal L12
  constraint vertical L13
  constraint horizontal L14
  constraint vertical L15
  constraint coincident L5.start L12
  constraint coincident L15 L16.start
  constraint coincident L13 L16.end
  constraint perpendicular L13 L16
  measures "d113" distance of L4 L14
  measures "d114" distance of L9 L13
  measures "d115" distance of L5 L15
  measures "d116" distance of L11 L16
sketch "bottom" plane through (0, -0.3, 0) normal (0, 1, 0) x (-1, 0, 0) in component "bottom shell"
  line L0 (-28, -1.7) -> (-1, -1.7)
  line L1 (-1, -1.7) -> (-1, 4.8)
  line L2 (-1, 4.8) -> (-28, 4.8)
  line L3 (-28, 4.8) -> (-28, -1.7)
  line L4 (-12.8, 6.3) -> (-12.8, 0.3) construction
  line L5 (-20.8, 6.3) -> (-20.8, 0.3) construction
  line L6 (-12.8, 0.3) -> (-20.8, 0.3) construction
  line L7 (-12.8, 3) -> (-20.8, 3) construction
  line L8 (-21.1, 6.3) -> (-12.5, 6.3)
  line L9 (-12.5, 6.3) -> (-12.5, 0)
  line L10 (-12.5, 0) -> (-21.1, 0)
  line L11 (-21.1, 0) -> (-21.1, 6.3)
  line L12 (-21.1, 3.3) -> (-12.5, 3.3)
  dimension "d117" = 0.3
  dimension "d118" = 0.3
  dimension "d119" = 0.3
  dimension "d120" = 0.3
  constraint horizontal L8
  constraint vertical L9
  constraint horizontal L10
  constraint vertical L11
  constraint coincident L5.start L8
  constraint coincident L11 L12.start
  constraint coincident L9 L12.end
  constraint perpendicular L9 L12
  measures "d117" distance of L6 L10
  measures "d118" distance of L4 L9
  measures "d119" distance of L5 L11
  measures "d120" distance of L7 L12
sketch "top" plane through (0, 39.3, 0) normal (0, -1, 0) x (1, 0, 0) in component "bottom shell"
  line L0 (1, -1.7) -> (28, -1.7)
  line L1 (28, -1.7) -> (28, 4.8)
  line L2 (28, 4.8) -> (1, 4.8)
  line L3 (1, 4.8) -> (1, -1.7)
  line L4 (14.8, 6.3) -> (14.8, 0.3) construction
  line L5 (14.8, 3) -> (10, 3) construction
  line L6 (10, 0.3) -> (14.8, 0.3) construction
  line L7 (10, 6.3) -> (10, 0.3) construction
  line L8 (15.1, 6.3) -> (9.7, 6.3)
  line L9 (9.7, 6.3) -> (9.7, 0)
  line L10 (9.7, 0) -> (15.1, 0)
  line L11 (15.1, 0) -> (15.1, 6.3)
  line L12 (15.1, 3.3) -> (9.7, 3.3)
  dimension "d121" = 0.3
  dimension "d122" = 0.3
  dimension "d123" = 0.3
  dimension "d124" = 0.3
  constraint horizontal L8
  constraint vertical L9
  constraint horizontal L10
  constraint vertical L11
  constraint coincident L4.start L8
  constraint coincident L11 L12.start
  constraint coincident L9 L12.end
  constraint perpendicular L9 L12
  measures "d121" distance of L5 L12
  measures "d122" distance of L6 L10
  measures "d123" distance of L4 L11
  measures "d124" distance of L7 L9
sketch "right" plane through (29.3, 0, 0) normal (-1, 0, 0) x (0, -1, 0) in component "bottom shell"
  line L0 (-38, -1.7) -> (-1, -1.7)
  line L1 (-1, -1.7) -> (-1, 4.8)
  line L2 (-1, 4.8) -> (-38, 4.8)
  line L3 (-38, 4.8) -> (-38, -1.7)
  line L4 (-11.7, 6.3) -> (-11.7, 0.3) construction
  line L5 (-11.7, 0.3) -> (-3.7, 0.3) construction
  line L6 (-3.7, 6.3) -> (-3.7, 0.3) construction
  line L7 (-3.7, 0.3) -> (-3.7, 2.7374)
  line L8 (-3.7, 2.7374) -> (-3.7, 3)
  line L9 (-3.7, 3) -> (-3.7, 4.8) construction
  line L10 (-3.7, 4.8) -> (-3.7, 6.3) construction
  line L11 (-3.7, 3) -> (-11.7, 3) construction
  line L12 (-3.4, 6.3) -> (-12, 6.3)
  line L13 (-12, 6.3) -> (-12, 0)
  line L14 (-12, 0) -> (-3.4, 0)
  line L15 (-3.4, 0) -> (-3.4, 6.3)
  line L16 (-3.4, 2.7) -> (-12, 2.7)
  dimension "d125" = 0.3
  dimension "d126" = 0.3
  dimension "d127" = 0.3
  dimension "d128" = 0.3
  constraint horizontal L12
  constraint vertical L13
  constraint horizontal L14
  constraint vertical L15
  constraint coincident L4.start L12
  constraint coincident L15 L16.start
  constraint coincident L13 L16.end
  constraint perpendicular L13 L16
  measures "d125" distance of L6 L15
  measures "d126" distance of L5 L14
  measures "d127" distance of L4 L13
  measures "d128" distance of L11 L16
extrude "Extrude5''" cut sketch "right" against normal blind 1 contours L13 L14 L15 L16 bodies 5 in component "bottom shell"
extrude "Extrude6''" cut sketch "right" against normal blind 0.2 contours L2 L13 L15 L16 bodies 5 in component "bottom shell"
extrude "Extrude7''" cut sketch "top" against normal blind 1 contours L9 L10 L11 L12 bodies 5 in component "bottom shell"
extrude "Extrude8''" cut sketch "top" against normal blind 0.2 contours L2 L9 L11 L12 bodies 5 in component "bottom shell"
extrude "Extrude9" cut sketch "left" against normal blind 1 contours L13 L14 L15 L16 bodies 5 in component "bottom shell"
extrude "Extrude10'" cut sketch "left" against normal blind 0.2 contours L2 L13 L15 L16 L19 bodies 5 in component "bottom shell"
extrude "Extrude11'" cut sketch "bottom" against normal blind 1 contours L9 L10 L11 L12 bodies 5 in component "bottom shell"
extrude "Extrude12'" cut sketch "bottom" against normal blind 0.2 contours L2 L9 L11 L12 bodies 5 in component "bottom shell"
fillet "Fillet2" radius 0.5 12 edges at (16.7298, 33.9453, -3.2) (19.3641, 34.6889, -3.2) (19.6405, 32.2774, -3.2) (18.8245, 30.4844, -3.2) (17.0113, 30.4406, -3.2) (15.001, 31.7031, -3.2) (22.3595, 32.2774, -3.2) (22.6359, 34.6889, -3.2) (25.2702, 33.9453, -3.2) (26.999, 31.7031, -3.2) (24.9887, 30.4406, -3.2) (23.1755, 30.4844, -3.2) on bodies 5 in component "bottom shell"
fillet "Fillet5" radius 0.5 9 edges at (26.193, 13.711, -3.2) (23.6642, 18.4912, -3.2) (18.9098, 20.9942, -3.2) (12.193, 20.9942, -3.2) (7.4014, 18.4912, -3.2) (4.9098, 13.711, -3.2) (4.9098, 27.711, -3.2) (7.4014, 32.4912, -3.2) (12.193, 34.9942, -3.2) on bodies 5 in component "bottom shell"
fillet "Fillet3'" radius 0.5 12 edges at (22.3595, 32.2774, -1.7) (22.6359, 34.6889, -1.7) (25.2702, 33.9453, -1.7) (26.999, 31.7031, -1.7) (24.9887, 30.4406, -1.7) (23.1755, 30.4844, -1.7) (15.001, 31.7031, -1.7) (16.7298, 33.9453, -1.7) (19.3641, 34.6889, -1.7) (19.6405, 32.2774, -1.7) (18.8245, 30.4844, -1.7) (17.0113, 30.4406, -1.7) on bodies 5 in component "bottom shell"
fillet "Fillet6" radius 0.5 9 edges at (26.193, 13.711, -1.7) (23.6642, 18.4912, -1.7) (18.9098, 20.9942, -1.7) (12.193, 20.9942, -1.7) (7.4014, 18.4912, -1.7) (4.9098, 13.711, -1.7) (4.9098, 27.711, -1.7) (7.4014, 32.4912, -1.7) (12.193, 34.9942, -1.7) on bodies 5 in component "bottom shell"
fillet "Fillet4" radius 0.5 8 edges at (29.3, 19.5, -1.7) (28.9192, 38.9192, -1.7) (14.5, 39.3, -1.7) (0.0808, 38.9192, -1.7) (-0.3, 19.5, -1.7) (0.0808, 0.0808, -1.7) (14.5, -0.3, -1.7) (28.9192, 0.0808, -1.7) on bodies 5 in component "bottom shell"
fillet "Fillet8" radius 2 4 edges at (12.4, 36.8, 6.3) (26.8, 7.7, 6.3) (16.8, 2.2, 6.3) (2.2, 7.7, 6.3) on bodies 6 in component "top shell"
fillet "Fillet9" radius 0.5 8 edges at (28.05, 11.7, 0.3) (28.05, 3.7, 0.3) (20.8, 0.95, 0.3) (12.8, 0.95, 0.3) (0.95, 3.7, 0.3) (0.95, 11.7, 0.3) (10, 38.05, 0.3) (14.8, 38.05, 0.3) on bodies 6 in component "top shell"
fillet "Fillet11" radius 0.5 8 edges at (14.8, 37.5768, 6.3) (10, 37.9387, 6.3) (27.05, 11.7, 6.3) (27.05, 3.7, 6.3) (20.8, 1.95, 6.3) (12.8, 1.95, 6.3) (1.95, 3.7, 6.3) (1.95, 11.7, 6.3) on bodies 6 in component "top shell"
fillet "Fillet12" radius 0.5 35 edges at (3.5085, 11.8712, 6.1766) (2.3771, 11.7, 5.1229) (2.2, 11.7, 2.55) (2.2, 11.5536, 0.4464) (2.2, 7.7, 0.3) (2.2, 3.8464, 0.4464) (2.2, 3.7, 2.55) (2.3771, 3.7, 5.1229) (3.5085, 3.5288, 6.1766) (12.6277, 3.5112, 6.1774) (12.8, 2.3771, 5.1229) (12.8, 2.2, 2.55) (12.9464, 2.2, 0.4464) (16.8, 2.2, 0.3) (20.6536, 2.2, 0.4464) (20.8, 2.2, 2.55) (20.8, 2.3771, 5.1229) (20.9723, 3.5112, 6.1774) (25.4915, 3.5288, 6.1766) (26.6229, 3.7, 5.1229) (26.8, 3.7, 2.55) (26.8, 3.8464, 0.4464) (26.8, 7.7, 0.3) (26.8, 11.5536, 0.4464) (26.8, 11.7, 2.55) (26.6229, 11.7, 5.1229) (25.4915, 11.8712, 6.1766) (14.8077, 36.0146, 5.8889) (14.8, 36.6229, 5.1229) (14.8, 36.8, 2.55) (14.6536, 36.8, 0.4464) (12.4, 36.8, 0.3) (10.1464, 36.8, 0.4464) (10, 36.8, 2.55) (10, 36.7436, 4.7718) on bodies 6 in component "top shell"
fillet "Fillet13" radius 0.5 20 edges at (-0.7821, 3.7, 1.7687) (-0.3481, 3.8464, 0.4464) (-0.3, 7.7, 0.3) (-0.3481, 11.5536, 0.4464) (-0.7821, 11.7, 1.7687) (10, 39.7821, 1.7687) (10.1464, 39.3481, 0.4464) (12.4, 39.3, 0.3) (14.6536, 39.3481, 0.4464) (14.8, 39.7821, 1.7687) (29.7821, 11.7, 1.7687) (29.3481, 11.5536, 0.4464) (29.3, 7.7, 0.3) (29.3481, 3.8464, 0.4464) (29.7821, 3.7, 1.7687) (20.8, -0.7821, 1.7687) (20.6536, -0.3481, 0.4464) (16.8, -0.3, 0.3) (12.9464, -0.3481, 0.4464) (12.8, -0.7821, 1.7687) on bodies 6 in component "top shell"
fillet "Fillet14" radius 0.5 29 edges at (10, 39.3, 5.3) (9.8536, 39.3, 6.1536) (5.25, 39.3, 6.3) (0.0808, 38.9192, 6.3) (-0.3, 25.1, 6.3) (-0.3, 11.8464, 6.1536) (-0.3, 11.7, 5.3) (18.15, 39.3, 6.3) (14.9464, 39.3, 6.1536) (14.8, 39.3, 5.3) (29.3, 11.7, 5.3) (29.3, 11.8464, 6.1536) (29.3, 25.1, 6.3) (28.9192, 38.9192, 6.3) (24.5, 39.3, 6.3) (20.8, -0.3, 5.3) (20.9464, -0.3, 6.1536) (24.65, -0.3, 6.3) (28.9192, 0.0808, 6.3) (29.3, 2.1, 6.3) (29.3, 3.5536, 6.1536) (29.3, 3.7, 5.3) (-0.3, 3.7, 5.3) (-0.3, 3.5536, 6.1536) (-0.3, 2.1, 6.3) (0.0808, 0.0808, 6.3) (6.65, -0.3, 6.3) (12.6536, -0.3, 6.1536) (12.8, -0.3, 5.3) on bodies 6 in component "top shell"
fillet "Fillet3''" radius 0.5 1 edges at (11.1353, 7.2768, 6.3) on bodies 6 in component "top shell"
fillet "Fillet4'" radius 0.3 6 edges at (15.8975, 19.9791, 6.3) (1.8975, 19.9791, 6.3) (3.2532, 28.0107, 6.3) (9.8001, 36.7023, 6.1998) (10.1683, 36.4625, 5.6219) (11.1249, 35.5969, 6.1344) on bodies 6 in component "top shell"
fillet "Fillet5'" radius 0.2 4 edges at (15.8975, 19.9791, 8.8) (14.194, 34.6398, 8.8) (1.8975, 19.9791, 8.8) (1.8975, 33.9791, 8.8) on bodies 6 in component "top shell"
fillet "Fillet7" radius 1 8 edges at (30.687, 40.687, 8.8) (14.5, 41.8, 8.8) (-1.6884, 40.6856, 8.8) (-2.8, 19.498, 8.8) (-1.687, -1.687, 8.8) (14.5, -2.8, 8.8) (30.687, -1.687, 8.8) (31.8, 19.5, 8.8) on bodies 6 in component "top shell"
sketch "label_outline" plane through (0, 0, 8.8) normal (0, 0, 1) x (-1, 0, 0) in component "top shell"
  circle A0 centre (-7, -32) radius 5.6729
  circle A1 centre (-21, -32) radius 7.5
  circle A2 centre (-21, -18) radius 5.6729
  circle A3 centre (-7, -18) radius 5.6729
  arc A4 (-30.8, -38) -> (-28, -40.8) centre (-28, -38) ccw
  line L0 (-28, -40.8) -> (-1, -40.8)
  arc A5 (-1, -40.8) -> (1.8, -37.997) centre (-1, -38) ccw
  line L1 (1.8, -37.997) -> (1.8, -1)
  arc A6 (1.8, -1) -> (-1, 1.8) centre (-1, -1) ccw
  line L2 (-1, 1.8) -> (-28, 1.8)
  arc A7 (-28, 1.8) -> (-30.8, -1) centre (-28, -1) ccw
  line L3 (-30.8, -1) -> (-30.8, -38)
  line L4 (1.8, -1) -> (1.8, -37.997)
  arc A8 (1.8, -1) -> (-1, 1.8) centre (-1, -1) ccw
  line L5 (-28, 1.8) -> (-1, 1.8)
  arc A9 (-28, 1.8) -> (-30.8, -1) centre (-28, -1) ccw
  line L6 (-30.8, -38) -> (-30.8, -1)
  circle A10 centre (-21, -18) radius 5.6729
  circle A11 centre (-7, -18) radius 5.6729
  circle A12 centre (-7, -32) radius 5.6729
  circle A13 centre (-21, -32) radius 7.5
  arc A14 (-30.8, -38) -> (-28, -40.8) centre (-28, -38) ccw
  line L7 (-1, -40.8) -> (-28, -40.8)
  arc A15 (-1, -40.8) -> (1.8, -37.997) centre (-1, -38) ccw